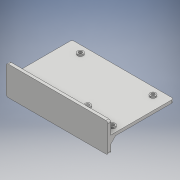
# Autodesk Inventor part: Eletronica - suporteArduino
Saved by Autodesk Inventor 2017 (Build 210142000, 142)
## iProperties
Created: 2020-10-10
Part Number: Eletronica - suporteArduino
Material: Generic
Document SubType Name: Modeling
Designer: ale
Density: 1 g/cm^3
Appearance: Default
Author: ale
Autodesk Inventor part; units mm, degrees
ref_plane "YZ Plane" through (0, 0, 0) normal (1, 0, 0) x (0, 1, 0)
ref_plane "XZ Plane" through (0, 0, 0) normal (0, 1, 0) x (-1, 0, 0)
ref_plane "XY Plane" through (0, 0, 0) normal (0, 0, 1) x (1, 0, 0)
sketch "Sketch1" plane through (0, 0, 0) normal (0, 0, 1) x (1, 0, 0)
  line L0 (-52.5, 32.5) -> (52.5, 32.5)
  line L1 (52.5, 32.5) -> (52.5, -32.5)
  line L2 (52.5, -32.5) -> (-52.5, -32.5)
  line L3 (-52.5, -32.5) -> (-52.5, 32.5)
  line L4 (-52.5, 32.5) -> (52.5, -32.5) construction
  line L5 (52.5, 32.5) -> (-52.5, -32.5) construction
  point P0 (0, 0)
  dimension "d0" = 105
  dimension "d1" = 65
  constraints: 12 end point, 2 midpoint, 2 parallel, 1 horizontal, 1 perpendicular
  measures "d0" distance of L1.end L2.end
  measures "d1" distance of L0.end L1.end
extrude "Extrusion1" add sketch "Sketch1" along normal blind 3
sketch "Sketch2" plane through (0, 0, 3) normal (0, 0, 1) x (1, 0, 0)
  line L0 (-50.8, 26.67) -> (50.8, 26.67)
  line L1 (50.8, 26.67) -> (50.8, -26.67)
  line L2 (50.8, -26.67) -> (-50.8, -26.67)
  line L3 (-50.8, -26.67) -> (-50.8, 26.67)
  line L4 (-50.8, 26.67) -> (50.8, -26.67) construction
  line L5 (50.8, 26.67) -> (-50.8, -26.67) construction
  line L6 (50.8, -24.13) -> (-50.8, -24.13)
  line L7 (-35.56, -26.67) -> (-35.56, 26.67)
  line L8 (50.8, 24.13) -> (-50.8, 24.13)
  circle A0 centre (-35.56, 24.13) radius 3
  line L9 (-36.83, -26.67) -> (-36.83, 26.67)
  circle A1 centre (-36.83, -24.13) radius 3
  line L10 (45.72, -26.67) -> (45.72, 26.67)
  circle A2 centre (45.72, -24.13) radius 3
  line L11 (15.24, -26.67) -> (15.24, 26.67)
  line L12 (50.8, -19.05) -> (-50.8, -19.05)
  circle A3 centre (15.24, -19.05) radius 3
  line L13 (39.37, -26.67) -> (39.37, 26.67)
  circle A4 centre (39.37, 24.13) radius 3
  point P0 (0, 0)
  dimension "d4" = 101.6
  dimension "d5" = 53.34
  dimension "d6" = 2.54
  dimension "d7" = 15.24
  dimension "d8" = 50.8
  dimension "d9" = 6
  dimension "d10" = 13.97
  dimension "d11" = 6
  dimension "d12" = 96.52
  dimension "d13" = 6
  dimension "d14" = 66.04
  dimension "d15" = 7.62
  dimension "d16" = 6
  dimension "d17" = 90.17
  dimension "d18" = 6
  constraints: 28 end point, 10 parallel, 10 point on line, 5 centre point, 2 midpoint, 1 horizontal, 1 perpendicular
  measures "d4" distance of L1.end L2.end
  measures "d5" distance of L0.end L1.end
  measures "d6" distance between parallel lines of L2 L6
  measures "d7" distance between parallel lines of L3 L7
  measures "d8" distance between parallel lines of L2 L8
  measures "d9" diameter of A0
  measures "d10" distance between parallel lines of L3 L9
  measures "d11" diameter of A1
  measures "d12" distance between parallel lines of L3 L10
  measures "d13" diameter of A2
  measures "d14" distance between parallel lines of L3 L11
  measures "d15" distance between parallel lines of L2 L12
  measures "d16" diameter of A3
  measures "d17" distance between parallel lines of L3 L13
  measures "d18" diameter of A4
extrude "Extrusion2" add sketch "Sketch2" along normal blind 1.5 contours L0 A0 | L9 L8 A0 L0 | L0 L7 L8 L9 | L0 A0 L8 L7 | L9 A0 L8 | L8 L7 A0 L9 | L8 A0 L7 | A4 L0 | L0 L13 L8 A4 | A1 L7 L6 L9 | L9 L6 A1 | L0 A4 L8 L13 | L8 L13 A4 | A3 L12 L11 | L11 L12 A3 | A1 L6 L7 | L12 L11 A3 | L9 L2 A1 L6 | L6 L7 L2 L9 | L8 A4 L13 | L12 A3 L11 | L6 A1 L2 L7 | L2 A1 | A2 L6 L10 | L10 L6 A2 | L6 L10 L2 A2 | L6 A2 L2 L10 | L2 A2
sketch "Sketch3" plane through (-35.56, 24.13, 4.5) normal (0, 0, 1) x (1, 0, 0)
  circle A0 centre (74.93, 0) radius 3 projected
  circle A1 centre (81.28, -48.26) radius 3 projected
  circle A2 centre (50.8, -43.18) radius 3 projected
  circle A3 centre (-1.27, -48.26) radius 3 projected
  point P0 (35.56, -24.13)
  point P1 (0, 0)
  constraints: 4 coincident
hole "Hole1" at (-35.56, 24.13, 4.5) at (39.37, 24.13, 4.5) at (45.72, -24.13, 4.5) at (15.24, -19.05, 4.5) at (-36.83, -24.13, 4.5) direction (0, 0, -1) diameter 3.5 end through all
sketch "Sketch4" plane through (-52.5, -32.5, 0) normal (0, -1, 0) x (1, 0, 0)
  line L0 (0, 0) -> (0, 3) projected
  line L1 (0, 1.5) -> (105, 1.5)
  line L2 (105, 0) -> (105, 3) projected
  line L3 (0, 16.5) -> (105, 16.5)
  line L4 (105, 16.5) -> (105, -13.5)
  line L5 (105, -13.5) -> (0, -13.5)
  line L6 (0, -13.5) -> (0, 16.5)
  line L7 (0, 16.5) -> (105, -13.5) construction
  line L8 (105, 16.5) -> (0, -13.5) construction
  point P0 (52.5, 0)
  point P1 (52.5, 1.5)
  dimension "d29" = 30
  constraints: 14 end point, 5 midpoint, 2 parallel, 1 horizontal, 1 perpendicular
  measures "d29" distance of L3.end L4.end
extrude "Extrusion3" add sketch "Sketch4" along normal blind 3
chamfer "Chamfer1" distance 5 angle 45 1 edges at (0, -32.5, 0)
fillet "Fillet1" radius 2 6 edges at (52.5, 32.5, 1.5) (52.5, -34, 16.5) (52.5, -34, -13.5) (-52.5, -34, -13.5) (-52.5, -34, 16.5) (-52.5, 32.5, 1.5)
body "Solid1"
